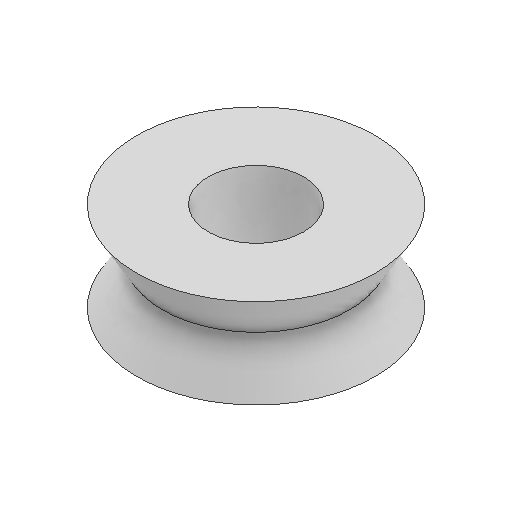
# Autodesk Inventor part: Spring Holder
Saved by Autodesk Inventor 2025 (Build 290162010, 162A)
## iProperties
Created: 2024-12-05
Part Number: Spring Holder
Material: Generic
Document SubType Name: Modeling
Designer: ALEXANDERNICHOLS
Density: 1 g/cm^3
Appearance: Default
Author: ALEXANDERNICHOLS
Autodesk Inventor part; units mm, degrees
ref_plane "YZ Plane" through (0, 0, 0) normal (1, 0, 0) x (0, 1, 0)
ref_plane "XZ Plane" through (0, 0, 0) normal (0, 1, 0) x (-1, 0, 0)
ref_plane "XY Plane" through (0, 0, 0) normal (0, 0, 1) x (1, 0, 0)
sketch "Sketch1" plane through (0, 0, 0) normal (0, 0, 1) x (1, 0, 0)
  line L0 (0, 0) -> (0, 3.81)
  line L1 (0, 3.81) -> (5.08, 3.81)
  line L2 (5.08, 3.81) -> (3.9801, 1.905)
  line L3 (3.9801, 1.905) -> (5.08, 0)
  line L4 (5.08, 0) -> (0, 0)
  line L5 (2.032, 0) -> (2.032, 3.81)
  point P0 (0, 1.905)
  dimension "d0" = 5.08
  dimension "d1" = 60
  dimension "d2" = 3.81
  dimension "d3" = 2.032
  constraints: 12 end point, 2 perpendicular, 2 point on line, 1 horizontal alignment, 1 midpoint, 1 parallel, 1 vertical, 1 vertical alignment
  measures "d0" distance of L0.end L1.end
  measures "d1" angle of L1 L2
  measures "d2" distance between parallel lines of L1 L4
  measures "d3" distance between parallel lines of L0 L5
revolve "Revolution1" add sketch "Sketch1" angle 360 about axis through (0, 0, 0) along (0, 1, 0) contours L5 L1 L2 L3 L4
body "Solid1"
